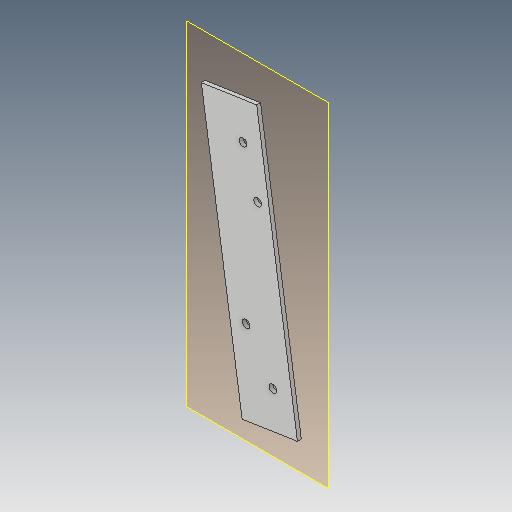
# Autodesk Inventor part: inside wall
Saved by Autodesk Inventor 2019 (Build 230136000, 136)
## iProperties
Created: 2019-10-13
Part Number: inside wall
Material: Generic
Document SubType Name: Modeling
Designer: ball
Density: 1 g/cm^3
Appearance: Default
Author: ball
Autodesk Inventor part; units mm, degrees
ref_plane "YZ Plane" through (0, 0, 0) normal (1, 0, 0) x (0, 1, 0)
ref_plane "XZ Plane" through (0, 0, 0) normal (0, 1, 0) x (-1, 0, 0)
ref_plane "XY Plane" through (0, 0, 0) normal (0, 0, 1) x (1, 0, 0)
ref_plane "Work Plane1" through (-0.0002, 0.0012, 0) normal (0, 0, 1) x (1, 0, 0)
sketch "Sketch1" plane through (-0.0002, 0.0012, 0) normal (0, 0, 1) x (1, 0, 0)
  circle A0 centre (0.0002, -0.0012) radius 6.3373 construction
  circle A1 centre (-43.983, 70.442) radius 6.3373 construction
  circle A2 centre (-25.2086, 253.0637) radius 6.3373 construction
  circle A3 centre (-49.0976, 326.5282) radius 6.3373 construction
  circle A4 centre (0.0002, -0.0012) radius 6.4135
  circle A5 centre (-43.983, 70.442) radius 6.4135
  circle A6 centre (-25.2086, 253.0637) radius 6.4135
  circle A7 centre (-49.0976, 326.5282) radius 6.4135
  circle A8 centre (-49.0976, 326.5282) radius 60.325 construction
  line L0 (-50.6844, -68.6254) -> (-117.7218, 377.2128)
  circle A9 centre (0.0002, -0.0012) radius 60.325 construction
  circle A10 centre (0.0002, -0.0012) radius 31.75 construction
  line L1 (40.367, -54.9346) -> (-26.6704, 390.9036)
  circle A11 centre (-49.0976, 326.5282) radius 31.75 construction
  line L2 (-50.6844, -68.6254) -> (40.367, -54.9346)
  line L3 (-117.7218, 377.2128) -> (-26.6704, 390.9036)
  line L4 (-72.5873, 132.8957) -> (-77.6428, 166.5178) construction
  point P0 (0.0002, -0.0012)
  dimension "d0" = 12.827
  dimension "d1" = 12.827
  dimension "d2" = 12.827
  dimension "d3" = 12.827
  dimension "d11" = 120.65
  dimension "d13" = 120.65
  dimension "d14" = 63.5
  dimension "d16" = 63.5
  constraints: 10 end point, 8 centre point, 8 coincident, 6 tangent, 2 perpendicular, 3 other
  measures "d0" diameter of A4
  measures "d1" diameter of A5
  measures "d2" diameter of A6
  measures "d3" diameter of A7
  measures "d11" diameter of A8
  measures "d13" diameter of A9
  measures "d14" diameter of A10
  measures "d16" diameter of A11
extrude "Extrusion1" add sketch "Sketch1" along normal blind 6.35
body "Solid1"
